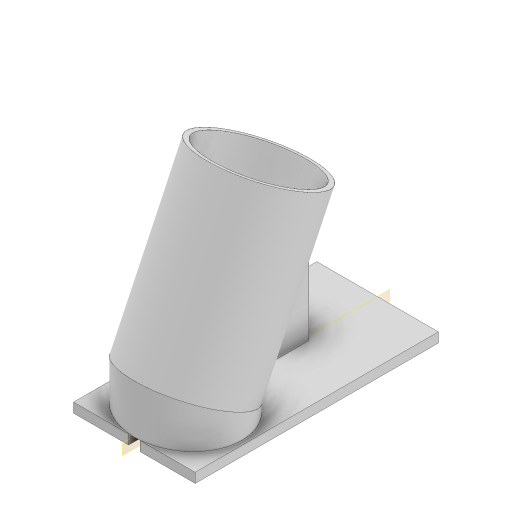
# Autodesk Inventor part: afirma_control_ps_move
Saved by Autodesk Inventor 2024 (Build 280153000, 153)
## iProperties
Created: 2023-06-20
Part Number: afirma_control_ps_move
Material: Generic
Document SubType Name: Modeling
Designer: ferna
Density: 1 g/cm^3
Appearance: Default
Author: ferna
Autodesk Inventor part; units mm, degrees
ref_plane "YZ Plane" through (0, 0, 0) normal (1, 0, 0) x (0, 1, 0)
ref_plane "XZ Plane" through (0, 0, 0) normal (0, 1, 0) x (-1, 0, 0)
ref_plane "XY Plane" through (0, 0, 0) normal (0, 0, 1) x (1, 0, 0)
sketch "Sketch1" plane through (0, 0, 0) normal (0, 1, 0) x (-1, 0, 0)
  line L0 (0, 0) -> (50, 0)
  line L1 (50, 0) -> (50, -100)
  line L2 (50, -100) -> (0, -100)
  line L3 (0, -100) -> (0, 0)
  dimension "d0" = 50
  dimension "d1" = 100
  constraints: 8 end point, 2 parallel, 1 horizontal, 1 perpendicular
  measures "d0" distance of L1.end L2.end
  measures "d1" distance of L0.end L1.end
extrude "Extrusion1" add sketch "Sketch1" along normal blind 4
ref_plane "Work Plane1" through (-25, 0, 0) normal (1, 0, 0) x (0, 0, -1)
sketch "Sketch2" plane through (-25, 0, 0) normal (1, 0, 0) x (0, 0, -1)
  line L0 (100, 4) -> (0, 4)
  line L1 (0, 4) -> (0, 24)
  line L2 (0, 24) -> (41.979161, 4)
  line L3 (20.989581, 14) -> (51.097108, 77.194437)
  line L4 (51.097108, 77.194437) -> (16.225312, 4)
  line L5 (0, 24) -> (30.107527, 87.194437)
  line L6 (30.107527, 87.194437) -> (51.097108, 77.194437)
  line L7 (51.097108, 77.194437) -> (72.086688, 67.194437)
  line L8 (72.086688, 67.194437) -> (41.979161, 4)
  line L9 (30.107527, 87.194437) -> (31.913082, 86.334222)
  line L10 (31.913082, 86.334222) -> (1.805555, 23.139785)
  line L11 (0, 24) -> (1.805555, 23.139785)
  line L12 (72.086688, 67.194437) -> (70.281133, 68.054652)
  line L13 (70.281133, 68.054652) -> (40.173606, 4.860215)
  line L14 (41.979161, 4) -> (40.173606, 4.860215)
  point P0 (0, 0)
  dimension "d5" = 20
  dimension "d6" = 46.5
  dimension "d7" = 2
  dimension "d8" = 2
  dimension "d10" = 70
  constraints: 28 end point, 7 point on line, 5 perpendicular, 2 collinear, 1 midpoint, 1 parallel, 1 vertical
  measures "d5" distance of L0.end L1.end
  measures "d6" distance of L1.end L2.end
  measures "d7" distance of L5.end L9.end
  measures "d8" distance of L7.end L12.end
  measures "d10" distance between parallel lines of L2 L6
revolve "Revolution1" add sketch "Sketch2" angle 360 about axis through (-25, 77.194437, -51.097108) along (0, -0.9027777, 0.4301075) contours L2 L13 L7 L8
sketch "Sketch3" plane through (0, 4, 0) normal (0, 1, 0) x (1, 0, 0)
  ellipse E0 centre (-25, 20.989581) end of major axis (-1.75, 20.989581) minor radius 20.989581
  ellipse E1 centre (-25, 20.989581) end of major axis (-3.75, 20.989581) minor radius 19.184025
  point P0 (0, 0)
  point P1 (-25, 41.979161)
  constraints: 1 vertical alignment
extrude "Extrusion2" add sketch "Sketch3" along normal up to surface contours E0 | E1 surface through (-25, 4.860215, -40.173606) normal (0, -0.9027777, 0.4301075)
sketch "Sketch4" plane through (0, 0, 0) normal (0, -1, 0) x (1, 0, 0)
  ellipse E0 centre (-25, -20.989581) end of major axis (-3.75, -20.989581) minor radius 19.184025
  circle A0 centre (-25, -20.989581) radius 9.307808
  point P0 (0, 0)
  constraints: 1 centre point, 1 coincident
extrude "Extrusion3" cut sketch "Sketch4" against normal blind 27.75 contours A0
sketch "Sketch5" plane through (0, 0, 0) normal (0, -1, 0) x (1, 0, 0)
  line L0 (-22.5659, 2.047168) -> (-22.5659, -12.366509)
  line L1 (-22.5659, -12.366509) -> (-27.37046, -12.366509)
  line L2 (-27.37046, -12.366509) -> (-27.37046, 2.047168)
  line L3 (-27.37046, 2.047168) -> (-22.5659, 2.047168)
  line L4 (-22.5659, 2.047168) -> (-27.37046, -12.366509) construction
  line L5 (-22.5659, -12.366509) -> (-27.37046, 2.047168) construction
  point P0 (0, 0)
  point P1 (-24.96818, -5.159671)
  constraints: 12 end point, 2 midpoint, 2 parallel, 1 perpendicular, 1 vertical
extrude "Extrusion4" cut sketch "Sketch5" against normal blind 4
sketch "Sketch7" plane through (0, 4, 0) normal (0, 1, 0) x (1, 0, 0)
  ellipse E0 centre (-25, 51.097108) end of major axis (-1.75, 51.097108) minor radius 20.989581
  ellipse E1 centre (-25, 20.989581) end of major axis (-1.75, 20.989581) minor radius 20.989581 (-25, 41.979161) -> (-27.37046, 0.109377) ccw
  ellipse E2 centre (-25, 20.989581) end of major axis (-1.75, 20.989581) minor radius 20.989581 (-22.5659, 0.115345) -> (-25, 41.979161) ccw
  ellipse E3 centre (-25, 51.097108) end of major axis (-3.75, 51.097108) minor radius 19.184025
  line L0 (-25, 72.086688) -> (-25, 51.097108)
  line L1 (-25, 51.097108) -> (-25.818578, 51.097108)
  circle A0 centre (-25, 41.979161) radius 1.5
  line L2 (-26.499364, 41.93547) -> (-26.499364, 70.23332)
  line L3 (-23.500636, 41.93547) -> (-23.500636, 70.23332)
  point P0 (0, 0)
  point P1 (-23.500636, 42.022853)
  point P2 (-26.499364, 42.022853)
  point P3 (-39.704707, 37.247954)
  point P4 (-10.295293, 37.247954)
  dimension "d17" = 3
  constraints: 8 end point, 3 vertical, 2 point on circle, 1 centre point, 1 coincident, 1 perpendicular, 1 vertical alignment, 8 other
  measures "d17" diameter of A0
extrude "Extrusion5" add sketch "Sketch7" along normal up to next contours A0 E2 E1 | A0 E2 E3 E1 | E3 L3 A0 L2 picked at (-25.193075, 42.473599)
body "Solid1"
